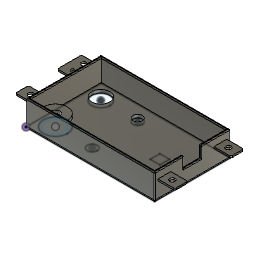
Modulator Famicom Box v7 (Autodesk Fusion 360 design; units mm, degrees)
Autodesk Fusion 360 part; units mm, degrees
sketch "Sketch2" plane through (0, 0, 0) normal (0, 0, 1) x (1, 0, 0)
  line L0 (0, 0) -> (80, 0)
  line L1 (80, 0) -> (80, 46.8)
  line L2 (80, 46.8) -> (0, 46.8)
  line L3 (0, 46.8) -> (0, 0)
  circle A0 centre (9, 9.3) radius 5.9
  circle A1 centre (9, 37.5) radius 5.6
  circle A2 centre (31.9, 37.5) radius 2.85
  circle A3 centre (31.9, 9.3) radius 3
  line L4 (56, 27.2) -> (62, 27.2)
  line L5 (62, 27.2) -> (62, 21.2)
  line L6 (62, 21.2) -> (56, 21.2)
  line L7 (56, 21.2) -> (56, 27.2)
  circle A4 centre (9, 9.3) radius 5.9
  circle A5 centre (9, 9.3) radius 7.4
  dimension "d1" = 80
  dimension "d2" = 46.8
  dimension "d3" = 11.8
  dimension "d4" = 9
  dimension "d5" = 9.3
  dimension "d6" = 11.2
  dimension "d7" = 9.3
  dimension "d8" = 9
  dimension "d9" = 5.7
  dimension "d10" = 31.9
  dimension "d11" = 9.3
  dimension "d12" = 6
  dimension "d13" = 9.3
  dimension "d14" = 31.9
  dimension "d15" = 6
  dimension "d16" = 6
  dimension "d17" = 18
  dimension "d18" = 21.2
  dimension "d123" = 11.8
  dimension "d124" = 14.8
  constraint horizontal L0
  constraint vertical L1
  constraint horizontal L2
  constraint vertical L3
  constraint coincident L0.start L3.end
  constraint horizontal L4
  constraint vertical L5
  constraint horizontal L6
  constraint vertical L7
  constraint concentric A0 A5
  measures "d1" distance of L0.start L0.end
  measures "d2" distance of L0.start L2.end
  measures "d3" diameter of A0
  measures "d4" distance of L3 A0.centre
  measures "d5" distance of L0 A0.centre
  measures "d6" diameter of A1
  measures "d7" distance of L2 A1.centre
  measures "d8" distance of L3 A1.centre
  measures "d9" diameter of A2
  measures "d10" distance of L3 A2.centre
  measures "d11" distance of L2 A2.centre
  measures "d12" diameter of A3
  measures "d13" distance of L0 A3.centre
  measures "d14" distance of L3 A3.centre
  measures "d15" distance of L4.start L4.end
  measures "d16" distance of L4.start L6.end
  measures "d17" distance of L1 L5
  measures "d18" distance of L0 L6
  measures "d123" diameter of A4
  measures "d124" diameter of A5
extrude "Extrude9" add sketch "Sketch2" along normal blind 5 contours A5 makes body 1
extrude "Extrude1" add sketch "Sketch2" along normal blind 2 separate body contours L0 L1 L2 L3 | A5 makes body 2
sketch "Sketch10" plane through (0, 0, 5) normal (0, 0, 1) x (-1, 0, 0)
  circle A0 centre (-9, -9.3) radius 5.9
  circle A1 centre (-9, -9.3) radius 7.4
  circle A2 centre (-9, -9.3) radius 2.8
  dimension "d127" = 5.6
  constraint concentric A0 A2
  measures "d127" diameter of A2
extrude "Extrude10" add sketch "Sketch10" along normal blind 2 separate body contours A0 | A1 makes body 3
sketch "Sketch3" plane through (0, 0, 2) normal (0, 0, 1) x (-1, 0, 0)
  circle A0 centre (-31.9, -9.3) radius 3
  circle A1 centre (-31.9, -37.5) radius 2.85
  circle A2 centre (-9, -37.5) radius 5.6
  line L0 (-62, -21.2) -> (-56, -21.2)
  line L1 (-56, -21.2) -> (-56, -27.2)
  line L2 (-56, -27.2) -> (-62, -27.2)
  line L3 (-62, -27.2) -> (-62, -21.2)
  circle A3 centre (-9, -9.3) radius 5.9
  line L4 (0, -46.8) -> (0, 0)
  line L5 (0, 0) -> (-80, 0)
  line L6 (-80, 0) -> (-80, -46.8)
  line L7 (-80, -46.8) -> (0, -46.8)
  line L8 (-1.5, -1.5) -> (-78.5, -1.5)
  line L9 (-78.5, -1.5) -> (-78.5, -45.3)
  line L10 (-78.5, -45.3) -> (-1.5, -45.3)
  line L11 (-1.5, -45.3) -> (-1.5, -1.5)
  line L12 (-1.5, -18.5) -> (-1.5, -28.3)
  line L13 (-78.5, -28.3) -> (-78.5, -18.5)
  dimension "d21" = 1.5
  dimension "d22" = 1.5
  dimension "d23" = 1.5
  dimension "d24" = 1.5
  constraint horizontal L8
  constraint vertical L9
  constraint horizontal L10
  constraint vertical L11
  constraint vertical L12
  constraint coincident L11 L12.end
  constraint vertical L13
  constraint coincident L9 L13.end
  measures "d21" distance of L4 L10.end
  measures "d22" distance of L6 L9
  measures "d23" distance of L7 L10
  measures "d24" distance of L5 L8
extrude "Extrude2" add sketch "Sketch3" along normal blind 13.5 contours L4 L5 L6 L7 bodies 2
sketch "Sketch4" plane through (80, 0, 0) normal (1, 0, 0) x (0, 1, 0)
  line L0 (0, 0) -> (46.8, 0)
  line L1 (46.8, 0) -> (46.8, 15.5)
  line L2 (46.8, 15.5) -> (0, 15.5)
  line L3 (0, 15.5) -> (0, 0)
  line L4 (36.8, 11) -> (44.8, 11)
  line L5 (44.8, 11) -> (44.8, 10)
  line L6 (44.8, 10) -> (36.8, 10)
  line L7 (36.8, 10) -> (36.8, 11)
  line L8 (2, 11) -> (10, 11)
  line L9 (10, 11) -> (10, 10)
  line L10 (10, 10) -> (2, 10)
  line L11 (2, 10) -> (2, 11)
  dimension "d34" = 10
  dimension "d35" = 2
  dimension "d36" = 8
  dimension "d37" = 1
  dimension "d38" = 2
  dimension "d39" = 8
  dimension "d40" = 10
  dimension "d108" = 42.8
  dimension "d122" = 1
  constraint horizontal L4
  constraint vertical L5
  constraint horizontal L6
  constraint vertical L7
  constraint horizontal L8
  constraint vertical L9
  constraint horizontal L10
  constraint vertical L11
  measures "d34" distance of L0 L5.end
  measures "d35" distance of L1 L4.end
  measures "d36" distance of L4.start L4.end
  measures "d37" distance of L4.start L6.end
  measures "d38" distance of L3 L8.start
  measures "d39" distance of L8.start L8.end
  measures "d40" distance of L0 L10
  measures "d108" distance of L5.end L10.end
  measures "d122" distance of L8 L10
extrude "Extrude3" add sketch "Sketch4" along normal blind 10.5 contours L4 L5 L6 L7 | L8 L9 L10 L11 bodies 2
fillet "Fillet1" radius 1 1 edges at (90.5, 44.8, 10.5) on bodies 2
fillet "Fillet2" radius 1 1 edges at (90.5, 36.8, 10.5) on bodies 2
fillet "Fillet3" radius 1 1 edges at (90.5, 10, 10.5) on bodies 2
fillet "Fillet4" radius 1 1 edges at (90.5, 2, 10.5) on bodies 2
sketch "Sketch5" plane through (0, 0, 11) normal (0, 0, 1) x (-1, 0, 0)
  arc A0 (-89.5, -36.8) -> (-90.5, -37.8) centre (-89.5, -37.8) ccw
  line L0 (-90.5, -37.8) -> (-90.5, -43.8)
  arc A1 (-90.5, -43.8) -> (-89.5, -44.8) centre (-89.5, -43.8) ccw
  line L1 (-89.5, -44.8) -> (-80, -44.8)
  line L2 (-80, -44.8) -> (-80, -36.8)
  line L3 (-80, -36.8) -> (-89.5, -36.8)
  circle A2 centre (-85, -40.8) radius 1.65
  dimension "d51" = 3.3
  dimension "d52" = 5.5
  dimension "d53" = 4
  measures "d51" diameter of A2
  measures "d52" distance of L0 A2.centre
  measures "d53" distance of L3 A2.centre
extrude "Extrude4" cut sketch "Sketch5" against normal blind 3 contours A2 bodies 2
sketch "Sketch6" plane through (0, 0, 11) normal (0, 0, 1) x (-1, 0, 0)
  arc A0 (-89.5, -2) -> (-90.5, -3) centre (-89.5, -3) ccw
  line L0 (-90.5, -3) -> (-90.5, -9)
  arc A1 (-90.5, -9) -> (-89.5, -10) centre (-89.5, -9) ccw
  line L1 (-89.5, -10) -> (-80, -10)
  line L2 (-80, -10) -> (-80, -2)
  line L3 (-80, -2) -> (-89.5, -2)
  circle A2 centre (-85, -6) radius 1.65
  dimension "d57" = 3.3
  dimension "d58" = 5.5
  dimension "d59" = 4
  measures "d57" diameter of A2
  measures "d58" distance of L0 A2.centre
  measures "d59" distance of L3 A2.centre
extrude "Extrude5" cut sketch "Sketch6" against normal blind 3 contours A2 bodies 2
fillet "Fillet5" radius 0.5 1 edges at (80, 0, 7.75) on bodies 2
fillet "Fillet6" radius 0.5 1 edges at (80, 46.8, 7.75) on bodies 2
fillet "Fillet7" radius 0.5 1 edges at (0, 46.8, 7.75) on bodies 2
fillet "Fillet8" radius 0.5 1 edges at (0, 0, 7.75) on bodies 2
fillet "Fillet9" radius 0.5 8 edges at (80, 23.4, 0) (79.8536, 46.6536, 0) (40, 46.8, 0) (0.1464, 46.6536, 0) (0, 23.4, 0) (0.1464, 0.1464, 0) (40, 0, 0) (79.8536, 0.1464, 0) on bodies 2
fillet "Fillet11" radius 0.5 1 edges at (40, 45.3, 15.5) on bodies 2
sketch "Sketch7" plane through (0, 0, 0) normal (-1, 0, 0) x (0, -1, 0)
  line L0 (-46.3, 15.5) -> (-46.3, 0.5)
  line L1 (-46.3, 0.5) -> (-0.5, 0.5)
  line L2 (-0.5, 0.5) -> (-0.5, 15.5)
  line L3 (-45, 11) -> (-30, 11)
  line L4 (-30, 11) -> (-30, 10)
  line L5 (-30, 10) -> (-45, 10)
  line L6 (-45, 10) -> (-45, 11)
  line L7 (-12, 11) -> (-4, 11)
  line L8 (-4, 11) -> (-4, 10)
  line L9 (-4, 10) -> (-12, 10)
  line L10 (-12, 10) -> (-12, 11)
  line L11 (-46.3, 0) -> (-0.5, 0)
  line L12 (-46.8, 15.5) -> (-46.8, 0.5)
  line L13 (0, 0.5) -> (0, 15.5)
  line L14 (-0.5, 15.5) -> (-46.3, 15.5)
  dimension "d78" = 1
  dimension "d79" = 1
  dimension "d80" = 8
  dimension "d82" = 10
  dimension "d83" = 10
  dimension "d84" = 15
  dimension "d85" = 1.8
  dimension "d86" = 4
  dimension "d109" = 41
  constraint horizontal L3
  constraint vertical L4
  constraint horizontal L5
  constraint vertical L6
  constraint horizontal L7
  constraint vertical L8
  constraint horizontal L9
  constraint vertical L10
  measures "d78" distance of L3.end L4.end
  measures "d79" distance of L7.end L8.end
  measures "d80" distance of L8 L10
  measures "d82" distance of L9 L11
  measures "d83" distance of L5 L11
  measures "d84" distance of L3.start L3.end
  measures "d85" distance of L6 L12
  measures "d86" distance of L8 L13
  measures "d109" distance of L5.end L8.end
extrude "Extrude6" add sketch "Sketch7" along normal blind 10.5 contours L3 L4 L5 L6 | L7 L8 L9 L10 bodies 2
sketch "Sketch8" plane through (0, 0, 11) normal (0, 0, 1) x (-1, 0, 0)
  line L0 (0, -4) -> (0, -12)
  line L1 (0, -12) -> (10.5, -12)
  line L2 (10.5, -12) -> (10.5, -4)
  line L3 (10.5, -4) -> (0, -4)
  circle A0 centre (5, -8) radius 1.65
  circle A1 centre (5, -41) radius 1.65
  line L4 (10.5, -30) -> (10.5, -45)
  line L5 (0, -45) -> (10.5, -45)
  circle A2 centre (5, -34) radius 1.15
  line L6 (0, -30) -> (10.5, -30)
  dimension "d89" = 3.3
  dimension "d90" = 4
  dimension "d91" = 5.5
  dimension "d92" = 3.3
  dimension "d93" = 5.5
  dimension "d94" = 4
  dimension "d95" = 2.3
  dimension "d96" = 5.5
  dimension "d97" = 4
  measures "d89" diameter of A0
  measures "d90" distance of L3 A0.centre
  measures "d91" distance of L2 A0.centre
  measures "d92" diameter of A1
  measures "d93" distance of A1.centre L4
  measures "d94" distance of A1.centre L5
  measures "d95" diameter of A2
  measures "d96" distance of L4 A2.centre
  measures "d97" distance of A2.centre L6
fillet "Fillet13" radius 1 1 edges at (-10.5, 4, 10.5) on bodies 2
fillet "Fillet14" radius 1 1 edges at (-10.5, 12, 10.5) on bodies 2
fillet "Fillet15" radius 1 1 edges at (-10.5, 30, 10.5) on bodies 2
fillet "Fillet16" radius 1 1 edges at (-10.5, 45, 10.5) on bodies 2
extrude "Extrude7" cut sketch "Sketch8" against normal blind 3 contours A0 | A1 | A2 bodies 2
sketch "Sketch9" plane through (0, 0, 15.5) normal (0, 0, 1) x (-1, 0, 0)
  line L0 (-78.5, -45.8) -> (-78.5, -1.5)
  line L1 (-78.5, -1.5) -> (-1.5, -1.5)
  line L2 (-1.5, -1.5) -> (-1.5, -45.8)
  line L3 (-1.5, -45.8) -> (-78.5, -45.8)
  arc A0 (0, -0.5) -> (-0.5, 0) centre (-0.5, -0.5) ccw
  line L4 (-0.5, 0) -> (-79.5, 0)
  arc A1 (-79.5, 0) -> (-80, -0.5) centre (-79.5, -0.5) ccw
  line L5 (-80, -0.5) -> (-80, -46.3)
  arc A2 (-80, -46.3) -> (-79.5, -46.8) centre (-79.5, -46.3) ccw
  line L6 (-79.5, -46.8) -> (-0.5, -46.8)
  arc A3 (-0.5, -46.8) -> (0, -46.3) centre (-0.5, -46.3) ccw
  line L7 (0, -46.3) -> (0, -0.5)
  line L8 (-78.5, -28.8) -> (-80, -28.8)
  line L9 (-80, -28.8) -> (-80, -18)
  line L10 (-80, -18) -> (-78.5, -18)
  line L11 (-78.5, -18) -> (-78.5, -28.8)
  dimension "d110" = 18
  dimension "d111" = 18
  constraint horizontal L8
  constraint vertical L9
  constraint horizontal L10
  constraint vertical L11
  constraint coincident L5 L9.end
  constraint coincident L0 L8.start
  measures "d110" distance of L4 L9.end
  measures "d111" distance of L6 L8.end
extrude "Extrude8" cut sketch "Sketch9" against normal blind 7 contours L0 L5 L8 L9 L10 L11 bodies 2
fillet "Fillet17" radius 0.5 9 edges at (80, 37.55, 15.5) (79.8536, 46.6536, 15.5) (40, 46.8, 15.5) (0.1464, 46.6536, 15.5) (0, 23.4, 15.5) (0.1464, 0.1464, 15.5) (40, 0, 15.5) (79.8536, 0.1464, 15.5) (80, 9.25, 15.5) on bodies 2
fillet "Fillet18" radius 0.5 10 edges at (80, 23.4, 8.5) (80, 18, 11.75) (79.8536, 18, 15.3536) (79, 18, 15.5) (79, 28.8, 15.5) (79.8536, 28.8, 15.3536) (80, 28.8, 11.75) (78.5, 23.4, 8.5) (78.5, 28.8, 12) (78.5, 18, 12) on bodies 2
fillet "Fillet19" radius 0.5 4 edges at (78.6464, 17.8536, 15.3536) (78.5, 9.5, 15.5) (40, 1.5, 15.5) (1.5, 23.65, 15.5) on bodies 2
fillet "Fillet20" radius 0.5 2 edges at (78.5, 37.55, 15.5) (78.6464, 28.9464, 15.3536) on bodies 2
extrude "Extrude11" add sketch "Sketch2" along normal blind 2 contours L4 L5 L6 L7 bodies 2
